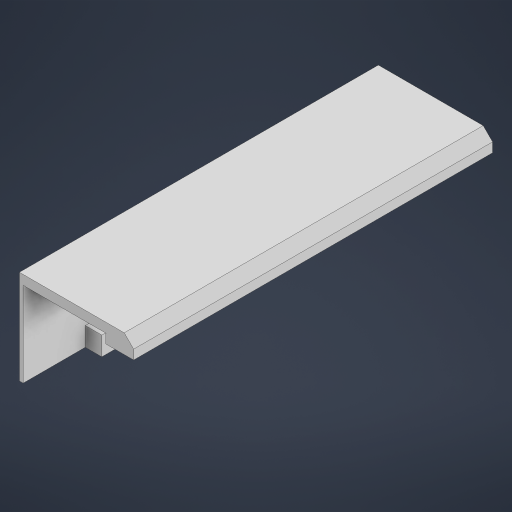
# Autodesk Inventor part: bumper belakang
Saved by Autodesk Inventor 2024.3 (Build 283343000, 343)
## iProperties
Created: 2025-06-14
Part Number: bumper belakang
Material: Generic
Document SubType Name: Modeling
Designer: Akbar Syihabuddin
Density: 1 g/cm^3
Appearance: Default
Author: Akbar Syihabuddin
Autodesk Inventor part; units mm, degrees
ref_plane "YZ Plane" through (0, 0, 0) normal (1, 0, 0) x (0, 1, 0)
ref_plane "XZ Plane" through (0, 0, 0) normal (0, 1, 0) x (-1, 0, 0)
ref_plane "XY Plane" through (0, 0, 0) normal (0, 0, 1) x (1, 0, 0)
sketch "Sketch1" plane through (0, 0, 0) normal (0, 1, 0) x (-1, 0, 0)
  line L0 (-32.3469, 68.4305) -> (-32.3469, -55.5695)
  line L1 (-17.6425, -88.9147) -> (-32.3469, -88.9147)
  line L2 (-32.3469, -88.9147) -> (-32.3469, -55.5695)
  line L3 (-32.3469, -55.5695) -> (-17.6425, -55.5695)
  line L4 (-17.6425, -55.5695) -> (-17.6425, -88.9147)
  line L5 (-27.3469, -55.5695) -> (-27.3469, 68.4305)
  line L6 (-32.3469, -55.5695) -> (-27.3469, -55.5695)
  line L7 (-27.3469, -55.5695) -> (-27.3469, 68.4305)
  line L8 (-27.3469, 68.4305) -> (-32.3469, 68.4305)
  line L9 (-32.3469, 68.4305) -> (-32.3469, -55.5695)
  line L10 (-32.3469, 68.4305) -> (-17.6425, 68.4305)
  line L11 (-17.6425, 68.4305) -> (-17.6425, 101.7757)
  line L12 (-17.6425, 101.7757) -> (-32.3469, 101.7757)
  line L13 (-32.3469, 101.7757) -> (-32.3469, 68.4305)
  point P0 (0, 0)
  point P1 (25.2053, -93.5695)
  constraints: 28 end point, 6 parallel, 3 horizontal, 3 perpendicular
extrude "Extrusion1" add sketch "Sketch1" along normal blind 10
chamfer "Chamfer1" distance 5 angle 45 3 edges at (32.3469, 10, -72.2421) (32.3469, 10, 6.4305) (32.3469, 10, 85.1031)
sketch "Sketch2" plane through (17.6425, 0, -88.9147) normal (-1, 0, 0) x (0, 0, 1)
  line L0 (0, 0) -> (0, 10) projected
  line L1 (33.3452, 0) -> (33.3452, 10) projected
  line L2 (0, 10) -> (33.3452, 10)
  line L3 (33.3452, 10) -> (33.3452, 5)
  line L4 (33.3452, 5) -> (0, 5)
  line L5 (0, 5) -> (0, 10)
  line L6 (157.3452, 10) -> (190.6905, 10) projected
  line L7 (157.3452, 0) -> (157.3452, 10) projected
  line L8 (190.6905, 10) -> (157.3452, 10)
  line L9 (157.3452, 10) -> (157.3452, 5)
  line L10 (157.3452, 5) -> (190.6905, 5)
  line L11 (190.6905, 5) -> (190.6905, 10)
  point P0 (88.9147, 0)
  dimension "d5" = 5
  constraints: 16 end point, 4 parallel, 2 horizontal, 2 midpoint, 2 perpendicular
  measures "d5" distance of L2.end L3.end
extrude "Extrusion2" add sketch "Sketch2" along normal blind 46
sketch "Sketch3" plane through (17.6425, 5, -88.9147) normal (0, -1, 0) x (1, 0, 0)
  line L0 (9.7044, 0) -> (-46, 0) projected
  line L1 (9.7044, 33.3452) -> (-46, 33.3452) projected
  line L2 (-46, 0) -> (-44, 0)
  line L3 (-44, 0) -> (-44, 33.3452)
  line L4 (-44, 33.3452) -> (-46, 33.3452)
  line L5 (-46, 33.3452) -> (-46, 0)
  line L6 (9.7044, 190.6905) -> (-46, 190.6905) projected
  line L7 (9.7044, 157.3452) -> (-46, 157.3452) projected
  line L8 (-46, 190.6905) -> (-45, 190.6905)
  line L9 (-45, 190.6905) -> (-45, 157.3452)
  line L10 (-45, 157.3452) -> (-46, 157.3452)
  line L11 (-46, 157.3452) -> (-46, 190.6905)
  point P0 (-17.6425, 88.9147)
  dimension "d8" = 2
  constraints: 16 end point, 4 parallel, 2 horizontal, 2 perpendicular, 2 point on line
  measures "d8" distance of L4.end L3.end
extrude "Extrusion3" add sketch "Sketch3" along normal blind 45
sketch "Sketch4" plane through (27.3469, 0, 68.4305) normal (0, 0, -1) x (-1, 0, 0)
  line L0 (0, 10) -> (55.7044, 10) projected
  line L1 (0, 0) -> (9.7517, 0)
  line L2 (9.7517, 0) -> (9.7517, 10)
  line L3 (9.7517, 10) -> (0, 10)
  line L4 (0, 10) -> (0, 0)
  line L5 (9.7517, 5) -> (55.7044, 5)
  line L6 (55.7044, 5) -> (55.7044, 10)
  line L7 (55.7044, 10) -> (9.7517, 10)
  line L8 (9.7517, 10) -> (9.7517, 5)
  line L9 (54.7044, 5) -> (54.7044, -40) projected
  line L10 (55.7044, 5) -> (54.7044, 5)
  line L11 (54.7044, 5) -> (54.7044, -40)
  line L12 (54.7044, -40) -> (55.7044, -40)
  line L13 (55.7044, -40) -> (55.7044, 5)
  point P0 (27.3469, 0)
  constraints: 24 end point, 6 parallel, 3 horizontal, 3 perpendicular, 1 midpoint, 1 point on line
extrude "Extrusion4" add sketch "Sketch4" along normal blind 150
sketch "Sketch5" plane through (-27.3575, 5, 101.7757) normal (1, 0, 0) x (0, 0, -1)
  line L0 (0, 0) -> (157.3452, 0) projected
  line L1 (190.6905, -45) -> (157.3452, -45) projected
  line L2 (0, 0) -> (157.3452, 0)
  line L3 (157.3452, 0) -> (157.3452, -45)
  line L4 (157.3452, -45) -> (0, -45)
  line L5 (0, -45) -> (0, 0)
  point P0 (101.7757, -5)
  constraints: 8 end point, 2 parallel, 1 horizontal, 1 perpendicular
extrude "Extrusion5" add sketch "Sketch5" along normal blind 1
sketch "Sketch6" plane through (-26.3575, 5, 101.7757) normal (1, 0, 0) x (0, 0, -1)
  line L0 (0, -45) -> (190.6905, -45) projected
  line L1 (190.6905, -45) -> (157.6905, -45)
  line L2 (0, -45) -> (33, -45)
  line L3 (33, -45) -> (157.6905, -45)
  line L4 (157.6905, -45) -> (157.6905, -35)
  line L5 (157.6905, -35) -> (33, -35)
  line L6 (33, -35) -> (33, -45)
  point P0 (101.7757, -5)
  dimension "d15" = 33
  dimension "d16" = 33
  dimension "d17" = 10
  constraints: 12 end point, 2 parallel, 2 point on line, 1 horizontal, 1 perpendicular
  measures "d15" distance of L0.end L1.end
  measures "d16" distance of L0.start L2.end
  measures "d17" distance of L4.end L3.end
extrude "Extrusion6" add sketch "Sketch6" along normal blind 8.786
sketch "Sketch7" plane through (-17.5715, 5, 101.7757) normal (1, 0, 0) x (0, 0, -1)
  line L0 (33, -45) -> (157.6905, -45) projected
  line L1 (95.3452, -45) -> (95.3452, -42.175)
  line L2 (95.3452, -42.175) -> (50.3452, -42.175)
  line L3 (95.3452, -42.175) -> (140.3452, -42.175)
  circle A0 centre (50.3452, -42.175) radius 1.5
  circle A1 centre (140.3452, -42.175) radius 1.5
  point P0 (101.7757, -5)
  dimension "d20" = 2.825
  dimension "d21" = 45
  dimension "d22" = 45
  dimension "d23" = 3
  dimension "d24" = 3
  constraints: 6 end point, 2 centre point, 2 coincident, 1 horizontal, 1 midpoint, 1 parallel, 1 vertical
  measures "d20" distance of L1.start L1.end
  measures "d21" distance of L1.end L2.end
  measures "d22" distance of L1.end L3.end
  measures "d23" diameter of A0
  measures "d24" diameter of A1
extrude "Extrusion7" cut sketch "Sketch7" against normal blind 40
body "Solid1"
